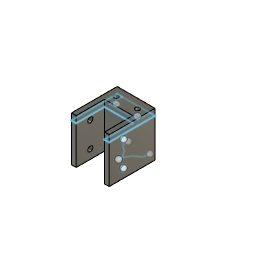
Servo back connector (Autodesk Fusion 360 design; units mm, degrees)
Autodesk Fusion 360 part; units mm, degrees
sketch "sketch 901" plane through (0, -26.35, 5.7) normal (0, 0, 1) x (1, 0, 0)
  circle A0 centre (-11.25, -16.9) radius 2.3
  circle A1 centre (11.25, -16.9) radius 2.3
  line L0 (15, -25.65) -> (15, -55.65)
  line L1 (15, -55.65) -> (20, -55.65)
  line L2 (20, -55.65) -> (20, -25.65)
  line L3 (20, -7.113) -> (20, -25.65)
  line L4 (20, -7.113) -> (14.5, -7.113)
  line L5 (-14.5, -7.113) -> (14.5, -7.113)
  line L6 (-20, -7.113) -> (-14.5, -7.113)
  line L7 (-20, -25.65) -> (-20, -7.113)
  line L8 (-20, -55.65) -> (-20, -25.65)
  line L9 (-15, -55.65) -> (-20, -55.65)
  line L10 (-15, -25.65) -> (-15, -55.65)
  line L11 (15, -25.65) -> (-15, -25.65)
extrude "Extrude1" add sketch "sketch 901" along normal blind 6.3 from surface at 0.5
sketch "sketch 849" plane through (0, -26.35, 5.7) normal (0, 0, 1) x (1, 0, 0)
  line L0 (20, -7.113) -> (14.8, -7.113)
  line L1 (14.8, -7.113) -> (14.8, -20.45)
  line L2 (14.8, -20.45) -> (-14.8, -20.45)
  line L3 (-14.8, -20.45) -> (-14.8, -7.113)
  line L4 (-20, -7.113) -> (-14.8, -7.113)
  line L5 (-20, -25.65) -> (-20, -7.113)
  line L6 (-20, -55.65) -> (-20, -25.65)
  line L7 (-15, -55.65) -> (-20, -55.65)
  line L8 (-15, -25.65) -> (-15, -55.65)
  line L9 (15, -25.65) -> (-15, -25.65)
  line L10 (15, -25.65) -> (15, -55.65)
  line L11 (15, -55.65) -> (20, -55.65)
  line L12 (20, -55.65) -> (20, -25.65)
  line L13 (20, -7.113) -> (20, -25.65)
extrude "Extrude2" add sketch "sketch 849" along normal up to surface (6.8 mm away) and the other way up to surface (17 mm away)
mirror "Mirror1" about plane through (0, -26.35, -11.3) normal (0, 0, 1) of bodies 1 merged
sketch "sketch 829" plane through (0, -56.2513, -35.1) normal (0, 0, -1) x (1, 0, 0)
  spline S0 degree 5 poles (0, -4.2513) (-0.0007, -4.475) (-0.0194, -4.9331) (-0.0988, -5.6526) (-0.3039, -6.6712) (-0.7042, -8.0109) (-1.2206, -9.3729) (-1.8257, -10.7093) (-2.4971, -11.9748) (-3.2254, -13.1353) (-4.0098, -14.1695) (-4.8521, -15.0698) (-5.7503, -15.8439) (-6.6936, -16.5155) (-7.6542, -17.1275) (-8.5918, -17.7363) (-9.4611, -18.4024) (-10.2186, -19.1834) (-10.8303, -20.125) (-11.2762, -21.2553) (-11.5457, -22.5903) (-11.6174, -23.8279) (-11.5901, -24.8522) (-11.536, -25.5778) (-11.5, -25.9513) knots 0 0 0 0 0 0 0.05 0.1 0.15 0.2 0.25 0.3 0.35 0.4 0.45 0.5 0.55 0.6 0.65 0.7 0.75 0.8 0.85 0.9 0.95 1 1 1 1 1 1
  spline S1 degree 5 poles (0.0067, -4.2513) (0.0074, -4.475) (0.0261, -4.9331) (0.1055, -5.6526) (0.3106, -6.6712) (0.7109, -8.0109) (1.2273, -9.3729) (1.8323, -10.7093) (2.5038, -11.9748) (3.2321, -13.1353) (4.0165, -14.1695) (4.8587, -15.0698) (5.757, -15.8439) (6.7003, -16.5155) (7.6609, -17.1275) (8.5984, -17.7363) (9.4678, -18.4024) (10.2253, -19.1834) (10.837, -20.125) (11.2828, -21.2553) (11.5524, -22.5903) (11.6241, -23.8279) (11.5968, -24.8522) (11.5427, -25.5778) (11.5067, -25.9513) knots 0 0 0 0 0 0 0.05 0.1 0.15 0.2 0.25 0.3 0.35 0.4 0.45 0.5 0.55 0.6 0.65 0.7 0.75 0.8 0.85 0.9 0.95 1 1 1 1 1 1
pipe "Pipe1" cut square section size 3 path "sketch 829" along S0
pipe "Pipe2" cut square section size 3 path "sketch 829" along S1
sketch "sketch 811" plane through (20, -56.2513, -11.3) normal (1, 0, 0) x (0, 1, 0)
  circle A0 centre (-10.7487, -14.3) radius 2.65
  circle A1 centre (-10.7487, 12.3) radius 2.65
extrude "Extrude3" cut sketch "sketch 811" against normal up to surface (5 mm away)
mirror "Mirror2" about plane through (0, -57.7315, -11.3) normal (1, 0, 0) of "Extrude3"
